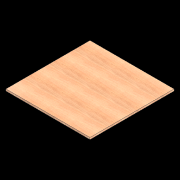
# Autodesk Inventor part: Floor
Saved by Autodesk Inventor 2022 (Build 260153000, 153)
## iProperties
Created: 2022-03-01
Part Number: Floor
Material: Wood (Birch)
Document SubType Name: Modeling
Designer: tandu
Density: 0.55 g/cm^3
Appearance: Birch - Natural Polished
Author: tandu
Autodesk Inventor part; units mm, degrees
ref_plane "YZ Plane" through (0, 0, 0) normal (1, 0, 0) x (0, 1, 0)
ref_plane "XZ Plane" through (0, 0, 0) normal (0, 1, 0) x (-1, 0, 0)
ref_plane "XY Plane" through (0, 0, 0) normal (0, 0, 1) x (1, 0, 0)
sketch "Sketch1" plane through (0, 0, 0) normal (0, 1, 0) x (-1, 0, 0)
  line L0 (-431.8, 431.8) -> (431.8, 431.8)
  line L1 (431.8, 431.8) -> (431.8, -431.8)
  line L2 (431.8, -431.8) -> (-431.8, -431.8)
  line L3 (-431.8, -431.8) -> (-431.8, 431.8)
  line L4 (-431.8, 431.8) -> (431.8, -431.8) construction
  line L5 (431.8, 431.8) -> (-431.8, -431.8) construction
  point P0 (0, 0)
  dimension "d1" = 863.6
  constraints: 12 end point, 2 midpoint, 2 parallel, 2 perpendicular, 1 horizontal
  measures "d1" distance of L1.end L2.end
extrude "Extrusion1" add sketch "Sketch1" along normal blind 19.05
equation "\"d1\" = BoxLength"
equation "\"BoxLength\" = 863.6"
body "Solid1"
